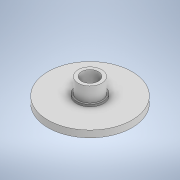
# Autodesk Inventor part: ShaibaNaPatron
Saved by Autodesk Inventor 2022 (Build 260153000, 153)
## iProperties
Created: 2023-08-16
Part Number: ShaibaNaPatron
Material: Generic
Document SubType Name: Modeling
Designer: Kippi
Density: 1 g/cm^3
Appearance: Default
Author: Kippi
Autodesk Inventor part; units mm, degrees
ref_plane "YZ Plane" through (0, 0, 0) normal (1, 0, 0) x (0, 1, 0)
ref_plane "XZ Plane" through (0, 0, 0) normal (0, 1, 0) x (-1, 0, 0)
ref_plane "XY Plane" through (0, 0, 0) normal (0, 0, 1) x (1, 0, 0)
sketch "Sketch1" plane through (0, 0, 0) normal (0, 1, 0) x (-1, 0, 0)
  circle A0 centre (0, 0) radius 125
  circle A1 centre (0, 0) radius 25
  dimension "d0" = 250
  dimension "d3" = 50
  constraints: 2 centre point, 2 coincident
  measures "d0" diameter of A0
  measures "d3" diameter of A1
extrude "Extrusion1" add sketch "Sketch1" along normal blind 20
sketch "Sketch2" plane through (0, 20, 0) normal (0, 1, 0) x (1, 0, 0)
  circle A0 centre (0, 0) radius 25 construction
  circle A1 centre (0, 0) radius 25
  circle A2 centre (0, 0) radius 35
  constraints: 2 centre point, 2 coincident, 1 concentric
extrude "Extrusion2" add sketch "Sketch2" along normal blind 50
sketch "Sketch3" plane through (0, 20, 0) normal (0, 1, 0) x (1, 0, 0)
  circle A0 centre (0, 0) radius 35 construction
  circle A1 centre (0, 0) radius 125 construction
  circle A2 centre (0, 0) radius 40
  circle A3 centre (0, 0) radius 35 construction
  circle A4 centre (0, 0) radius 35
  dimension "d6" = 5
  dimension "d7" = 80
  constraints: 2 centre point, 2 coincident, 1 concentric
  measures "d6" radial gap between concentric circles of A2 A0
  measures "d7" diameter of A2
extrude "Extrusion3" add sketch "Sketch3" along normal blind 6
body "Solid1"
